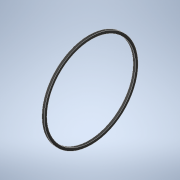
# Autodesk Inventor part: O-Ring_ID50mm_AD54mm
Saved by Autodesk Inventor 2021 (Build 250183000, 183)
## iProperties
Created: 2021-05-14
Part Number: O-Ring_ID50mm_AD54mm
Material: UHMW, Schwarz
Document SubType Name: Modeling
Designer: Michael
Density: 0.94 g/cm^3
Appearance: Glatt - Schwarz
Author: Michael
Autodesk Inventor part; units mm, degrees
ref_plane "YZ Plane" through (0, 0, 0) normal (1, 0, 0) x (0, 1, 0)
ref_plane "XZ Plane" through (0, 0, 0) normal (0, 1, 0) x (-1, 0, 0)
ref_plane "XY Plane" through (0, 0, 0) normal (0, 0, 1) x (1, 0, 0)
sketch "Skizze1" plane through (0, 0, 0) normal (0, 1, 0) x (-1, 0, 0)
  line L0 (0.6614, 26.5) -> (-0.6614, 26.5)
  line L1 (0.6614, 25) -> (-0.6614, 25)
  arc A0 (0.6614, 25) -> (0.6614, 26.5) centre (0, 25.75) ccw
  arc A1 (-0.6614, 26.5) -> (-0.6614, 25) centre (0, 25.75) ccw
  line L2 (1.4, 0) -> (-1.4, 0) projected
  point P0 (0, 0)
  dimension "d1" = 25.75
  dimension "d2" = 25
  dimension "d3" = 26.5
  constraints: 4 end point, 4 point on circle, 2 centre point, 2 horizontal
  measures "d1" distance of point (0, 0) A0.centre
  measures "d2" distance from line of point (0, 0) L1
  measures "d3" distance from line of point (0, 0) L0
revolve "Umdrehung1" add sketch "Skizze1" angle 360 about axis through (-10, 0, 0) along (1, 0, 0)
